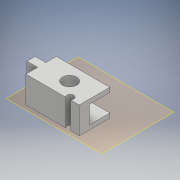
# Autodesk Inventor part: long selector
Saved by Autodesk Inventor 2017 (Build 210142000, 142)
## iProperties
Created: 2018-04-17
Part Number: long selector
Material: Generic
Document SubType Name: Modeling
Designer: RKL
Density: 1 g/cm^3
Appearance: Default
Author: RKL
Autodesk Inventor part; units mm, degrees
ref_plane "YZ Plane" through (0, 0, 0) normal (1, 0, 0) x (0, 1, 0)
ref_plane "XZ Plane" through (0, 0, 0) normal (0, 1, 0) x (-1, 0, 0)
ref_plane "XY Plane" through (0, 0, 0) normal (0, 0, 1) x (1, 0, 0)
ref_plane "Work Plane1" through (0, 0, 0) normal (0, 0, 1) x (1, 0, 0)
sketch "Sketch1" plane through (0, 0, 0) normal (0, 0, 1) x (1, 0, 0)
  circle A0 centre (7, -8.8957) radius 4 projected
  circle A1 centre (-2.136, 8.8957) radius 4 construction
  line L0 (-8.905, 18.405) -> (-8.905, 11.3957) construction
  line L1 (-8.905, 11.3957) -> (-14.905, 11.3957) construction
  line L2 (-14.905, 11.3957) -> (-14.905, 6.3957) construction
  line L3 (-14.905, 6.3957) -> (-8.905, 6.3957) construction
  line L4 (-8.905, 6.3957) -> (-8.905, -6.3957) construction
  line L5 (-8.905, -6.3957) -> (-14.905, -6.3957) construction
  line L6 (-14.905, -6.3957) -> (-14.905, -11.3957) construction
  line L7 (-14.905, -11.3957) -> (-8.905, -11.3957) construction
  line L8 (-8.905, -11.3957) -> (-8.905, -18.405) construction
  line L9 (-8.905, -18.405) -> (15, -18.405) construction
  circle A2 centre (15, -16.5) radius 1.905 construction
  line L10 (15, -18.405) -> (34, -18.405) construction
  line L11 (34, 18.405) -> (34, -18.405) construction
  line L12 (34, 18.405) -> (15, 18.405) construction
  circle A3 centre (15, 16.5) radius 1.905 construction
  line L13 (15, 18.405) -> (-8.905, 18.405) construction
  arc A4 (13.5995, 17.7914) -> (16.4005, 17.7914) centre (15, 16.5) ccw construction
  line L14 (13.5995, 17.7914) -> (-8.705, 17.7914) construction
  line L15 (-8.705, 17.7914) -> (-8.705, 11.1957) construction
  line L16 (-8.705, 11.1957) -> (-14.705, 11.1957) construction
  line L17 (-14.705, 11.1957) -> (-14.705, 6.5957) construction
  line L18 (-14.705, 6.5957) -> (-8.705, 6.5957) construction
  line L19 (-8.705, 6.5957) -> (-8.705, 0) construction
  line L20 (-8.705, 0) -> (21.295, 0) construction
  line L21 (21.295, 0) -> (21.295, 17.7914) construction
  line L22 (21.295, 17.7914) -> (16.4005, 17.7914) construction
  circle A5 centre (-2.136, 8.8957) radius 4 construction
  circle A6 centre (7, -8.8957) radius 4 construction
  line L23 (-14.705, -11.1957) -> (-8.705, -11.1957)
  line L24 (-8.705, -11.1957) -> (-8.705, -6.5957)
  line L25 (-8.705, -6.5957) -> (-14.705, -6.5957)
  line L26 (-14.705, -6.5957) -> (-14.705, -11.1957)
  line L27 (-8.705, -17.7914) -> (21.295, -17.7914)
  line L28 (21.295, -17.7914) -> (21.295, 0)
  line L29 (21.295, 0) -> (-8.705, 0)
  line L30 (-8.705, 0) -> (-8.705, -17.7914)
  point P0 (0, 0)
  point P1 (-8.705, -8.8957)
  dimension "d0" = 0.2
  constraints: 16 end point, 4 equal length, 4 parallel, 2 horizontal, 2 midpoint, 2 perpendicular, 1 horizontal alignment
  measures "d0" distance between parallel lines of L6 L26
extrude "Extrusion1" add sketch "Sketch1" along normal blind 15
sketch "Sketch2" plane through (0, 0, 15) normal (0, 0, 1) x (1, 0, 0)
  circle A0 centre (15, -16.5) radius 1.905 projected
  point P0 (0, 0)
extrude "Extrusion2" cut sketch "Sketch2" against normal through all
sketch "Sketch3" plane through (21.295, -17.7914, 0) normal (1, 0, 0) x (0, 0, -1)
  line L0 (0, 0) -> (0, 17.7914) construction
  line L1 (0, 17.7914) -> (-15, 17.7914) construction
  line L2 (-15, 0) -> (-15, 17.7914) construction
  line L3 (0, 0) -> (-15, 0) construction
  line L4 (-18.5, 17.7914) -> (-28.5, 17.7914) construction
  line L5 (-18.5, 29.7914) -> (-18.5, 17.7914) construction
  line L6 (-28.5, 29.7914) -> (-18.5, 29.7914) construction
  line L7 (-28.5, 17.7914) -> (-28.5, 29.7914) construction
  line L8 (-2.5, 5.7914) -> (-12.5, 5.7914)
  line L9 (-12.5, 5.7914) -> (-12.5, 17.7914)
  line L10 (-12.5, 17.7914) -> (-2.5, 17.7914)
  line L11 (-2.5, 17.7914) -> (-2.5, 5.7914)
  point P0 (0, 17.7914)
  point P1 (-7.5, 17.7914)
  constraints: 8 end point, 4 parallel, 2 midpoint, 1 horizontal, 1 perpendicular
extrude "Extrusion3" cut sketch "Sketch3" against normal blind 10
sketch "Sketch4" plane through (-8.705, 0, 0) normal (0, 1, 0) x (1, 0, 0)
  line L0 (30, -12.5) -> (20, -12.5) projected
  line L1 (20, -12.5) -> (20, -2.5) projected
  line L2 (20, -2.5) -> (30, -2.5) projected
  line L3 (30, 0) -> (30, -2.5) projected
  line L4 (30, 0) -> (0, 0) projected
  line L5 (0, 0) -> (0, -15) projected
  line L6 (30, -15) -> (0, -15) projected
  line L7 (30, -12.5) -> (30, -15) projected
  point P0 (8.705, 0)
extrude "Extrusion4" cut sketch "Sketch4" against normal blind 0.6
body "Solid1"
